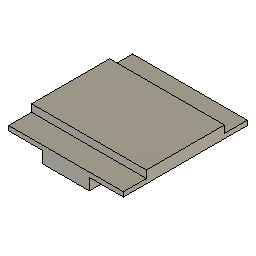
display_module (Autodesk Fusion 360 design; units mm, degrees)
part number: 2025-08-31-09-30-46-644
Autodesk Fusion 360 part; units mm, degrees
sketch "Sketch1" plane through (0, 0, 0) normal (0, 0, 1) x (1, 0, 0)
  line L0 (12.5, 13.5) -> (-12.5, 13.5)
  line L1 (-12.5, 13.5) -> (-12.5, -13.5)
  line L2 (-12.5, -13.5) -> (12.5, -13.5)
  line L3 (12.5, -13.5) -> (12.5, 13.5)
  line L4 (12.5, -13.5) -> (-12.5, 13.5) construction
  dimension "d1" = 25
  dimension "d2" = 27
  constraint horizontal L0
  constraint vertical L1
  constraint horizontal L2
  constraint vertical L3
  constraint midpoint origin L4
  measures "d1" distance of L0.start L0.end
  measures "d2" distance of L0.start L2.end
extrude "Extrude1" add sketch "Sketch1" along normal blind 1
sketch "Sketch2" plane through (0, 0, 0) normal (0, 0, -1) x (1, 0, 0)
  line L0 (12.5, -13.5) -> (12.5, 13.5)
  line L1 (12.5, 13.5) -> (-12.5, 13.5)
  line L2 (-12.5, 13.5) -> (-12.5, -13.5)
  line L3 (-12.5, -13.5) -> (12.5, -13.5)
  line L4 (-5.08, 10.96) -> (5.08, 10.96)
  line L5 (5.08, 10.96) -> (5.08, 13.5)
  line L6 (5.08, 13.5) -> (-5.08, 13.5)
  line L7 (-5.08, 13.5) -> (-5.08, 10.96)
  dimension "d5" = 2.54
  dimension "d6" = 10.16
  constraint horizontal L4
  constraint vertical L5
  constraint horizontal L6
  constraint vertical L7
  constraint midpoint L1 L6
  measures "d5" distance of L4.start L6.end
  measures "d6" distance of L4.start L4.end
extrude "Extrude2" add sketch "Sketch2" along normal blind 2.54 contours L1 L4 L5 L6 L7
sketch "Sketch3" plane through (0, 0, 1) normal (0, 0, 1) x (-1, 0, 0)
  line L0 (-12.5, 13.5) -> (-12.5, -13.5)
  line L1 (-12.5, -13.5) -> (12.5, -13.5)
  line L2 (12.5, -13.5) -> (12.5, 13.5)
  line L3 (12.5, 13.5) -> (-12.5, 13.5)
  line L4 (12.5, 8.5) -> (-12.5, 8.5)
  line L5 (-12.5, 8.5) -> (-12.5, -8.5)
  line L6 (-12.5, -8.5) -> (12.5, -8.5)
  line L7 (12.5, -8.5) -> (12.5, 8.5)
  line L8 (0, 8.5) -> (0, 13.5) construction
  dimension "d9" = 17
  dimension "d10" = 5
  constraint horizontal L4
  constraint vertical L5
  constraint horizontal L6
  constraint vertical L7
  constraint coincident L0 L5.end
  constraint coincident L2 L4.start
  constraint midpoint L4 L8.start
  constraint midpoint L3 L8.end
  measures "d9" distance of L4.start L6.end
  measures "d10" distance of L8.start L8.end
extrude "Extrude3" add sketch "Sketch3" along normal blind 1.6 contours L0 L2 L4 L5 L6 L7
